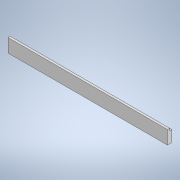
# Autodesk Inventor part: front beam
Saved by Autodesk Inventor 2020 (Build 240168000, 168)
## iProperties
Created: 2020-05-09
Part Number: front beam
Material: Generic
Document SubType Name: Modeling
Designer: kolbe
Density: 1 g/cm^3
Appearance: Default
Author: kolbe
Autodesk Inventor part; units mm, degrees
ref_plane "YZ Plane" through (0, 0, 0) normal (1, 0, 0) x (0, 1, 0)
ref_plane "XZ Plane" through (0, 0, 0) normal (0, 1, 0) x (-1, 0, 0)
ref_plane "XY Plane" through (0, 0, 0) normal (0, 0, 1) x (1, 0, 0)
sketch "Sketch1" plane through (0, 0, 0) normal (1, 0, 0) x (0, 1, 0)
  line L0 (0, 0) -> (0, -25.4)
  line L1 (0, -25.4) -> (63.5, -25.4)
  line L2 (63.5, -25.4) -> (63.5, -12.7)
  line L3 (63.5, -12.7) -> (76.2, -12.7)
  line L4 (76.2, -12.7) -> (76.2, 0)
  line L5 (76.2, 0) -> (0, 0)
  dimension "d0" = 25.4
  dimension "d1" = 63.5
  dimension "d2" = 12.7
  dimension "d3" = 12.7
  dimension "d4" = 12.7
  constraints: 12 end point, 3 perpendicular, 1 horizontal, 1 vertical
  measures "d0" distance of L0.start L0.end
  measures "d1" distance of L0.end L1.end
  measures "d2" distance of L1.end L2.end
  measures "d3" distance of L2.end L3.end
  measures "d4" distance of L3.end L4.end
extrude "Extrusion1" add sketch "Sketch1" along normal mid plane 901.7
body "Solid1"
